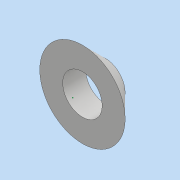
# Autodesk Inventor part: stożek
Saved by Autodesk Inventor 2017 (Build 210142000, 142)
## iProperties
Created: 2017-11-03
Part Number: stożek
Material: Ogólny
Document SubType Name: Modeling
Designer: Kuba01
Density: 1 g/cm^3
Appearance: Domyślna
Author: Kuba01
Autodesk Inventor part; units mm, degrees
ref_plane "YZ Plane" through (0, 0, 0) normal (1, 0, 0) x (0, 1, 0)
ref_plane "XZ Plane" through (0, 0, 0) normal (0, 1, 0) x (-1, 0, 0)
ref_plane "XY Plane" through (0, 0, 0) normal (0, 0, 1) x (1, 0, 0)
sketch "Szkic1" plane through (0, 0, 0) normal (0, 0, 1) x (1, 0, 0)
  point P0 (0, 0)
sketch "Szkic2" plane through (0, 0, 0) normal (0, 0, 1) x (1, 0, 0)
  line L0 (-13.5416, 0) -> (-13.4291, 0)
  line L1 (1.4961, 41.2359) -> (1.4961, -21.0278)
  line L2 (-13.4291, 24.1496) -> (-31.5039, 6.0748)
  line L3 (-13.4291, 0) -> (0, 0)
  line L4 (-13.4291, 24.1496) -> (-13.4291, 6.0748)
  line L5 (-24.5039, 13.0748) -> (-24.5039, 6.0748)
  line L6 (-31.5039, 6.0748) -> (-13.4291, 6.0748)
  dimension "d1" = 52
  dimension "d2" = 45
  dimension "d3" = 29.8504
  dimension "d6" = 7
  dimension "d7" = 7
  dimension "d8" = 18.0748
  constraints: 14 end point, 3 perpendicular, 2 point on line, 1 horizontal, 1 vertical
  measures "d1" diameter of L5 L1
  measures "d2" angle of L3 L2
  measures "d3" diameter of L4 L1
  measures "d6" distance of L5.end L5.start
  measures "d7" distance from line of L6 L5.start
  measures "d8" distance from line of L2.start L6
revolve "Obrót1" add sketch "Szkic2" angle 360 about axis through (1.4961, 41.2359, 0) along (0, -1, 0)
sketch "Szkic3" plane through (1.4961, 6.0748, 0) normal (0, -1, 0) x (1, 0, 0)
  circle A0 centre (0, 0) radius 14.9252 projected
  circle A1 centre (0, 0) radius 33 projected
  circle A2 centre (0, 0) radius 15.25
  point P0 (-1.4961, 0)
  dimension "d9" = 30.5
  constraints: 1 centre point, 1 coincident
  measures "d9" diameter of A2
extrude "Wyciągnięcie proste1" cut sketch "Szkic3" against normal through all contours A0 | A2
